Autodesk Fusion 360 part; units mm, degrees
note: some values were not read from the file. Chosen so that the rebuilt part matches the saved one: which bodies a step acts on. Set by a fixed rule: which sketch regions a step uses.
(part 4 of 6)
  spline S102 degree 5 poles (-98.784, -81.1032) (-98.7935, -81.0533) (-98.8123, -80.9538) (-98.8398, -80.8052) (-98.8751, -80.6086) (-98.9171, -80.3651) (-98.9568, -80.1241) (-98.9941, -79.8857) (-99.0292, -79.6497) (-99.062, -79.4165) (-99.0924, -79.1859) (-99.1207, -78.9582) (-99.1467, -78.7334) (-99.1706, -78.5115) (-99.1924, -78.2927) (-99.2121, -78.077) (-99.2297, -77.8644) (-99.2453, -77.6552) (-99.2589, -77.4492) (-99.2705, -77.2468) (-99.2802, -77.048) (-99.2881, -76.8529) (-99.2941, -76.6618) (-99.2983, -76.4747) (-99.3008, -76.2918) (-99.3016, -76.113) (-99.301, -75.9732) (-99.2997, -75.8702) (-99.2986, -75.8023) (-99.2979, -75.7686) knots 0 0 0 0 0 0 0.04 0.08 0.12 0.16 0.2 0.24 0.28 0.32 0.36 0.4 0.44 0.48 0.52 0.56 0.6 0.64 0.68 0.72 0.76 0.8 0.84 0.88 0.92 0.96 1 1 1 1 1 1
  arc A102 (-99.2979, -75.7686) -> (-97.2516, -81.4429) centre (-96.9333, -78.1219) ccw
  spline S103 degree 5 poles (-97.2516, -81.4429) (-97.2219, -81.4017) (-97.1628, -81.3194) (-97.0751, -81.1964) (-96.96, -81.0331) (-96.8191, -80.8302) (-96.6813, -80.6286) (-96.5466, -80.4283) (-96.4151, -80.2293) (-96.2868, -80.0317) (-96.1618, -79.8356) (-96.0399, -79.6412) (-95.9213, -79.4484) (-95.8059, -79.2574) (-95.6937, -79.0683) (-95.5847, -78.8812) (-95.4789, -78.696) (-95.3763, -78.5129) (-95.277, -78.332) (-95.1809, -78.1534) (-95.088, -77.9773) (-94.9985, -77.8039) (-94.9123, -77.6332) (-94.8294, -77.4655) (-94.7498, -77.3007) (-94.6735, -77.139) (-94.615, -77.012) (-94.5726, -76.9181) (-94.545, -76.8561) (-94.5313, -76.8253) knots 0 0 0 0 0 0 0.04 0.08 0.12 0.16 0.2 0.24 0.28 0.32 0.36 0.4 0.44 0.48 0.52 0.56 0.6 0.64 0.68 0.72 0.76 0.8 0.84 0.88 0.92 0.96 1 1 1 1 1 1
  arc A103 (-91.6439, -82.4317) -> (-94.5313, -76.8253) centre (-94.7025, -80.4602) ccw
  spline S104 degree 5 poles (-91.6439, -82.4317) (-91.6577, -82.3828) (-91.6851, -82.2853) (-91.7255, -82.1397) (-91.7778, -81.9469) (-91.8408, -81.708) (-91.9013, -81.4714) (-91.9594, -81.2371) (-92.0149, -81.0051) (-92.0678, -80.7756) (-92.1183, -80.5486) (-92.1663, -80.3242) (-92.2118, -80.1025) (-92.255, -79.8836) (-92.2957, -79.6675) (-92.3341, -79.4543) (-92.3702, -79.2441) (-92.404, -79.037) (-92.4355, -78.8331) (-92.4647, -78.6324) (-92.4917, -78.4351) (-92.5165, -78.2415) (-92.5391, -78.0517) (-92.5596, -77.8657) (-92.5781, -77.6836) (-92.5945, -77.5056) (-92.606, -77.3663) (-92.6138, -77.2635) (-92.6186, -77.1958) (-92.6208, -77.1622) knots 0 0 0 0 0 0 0.04 0.08 0.12 0.16 0.2 0.24 0.28 0.32 0.36 0.4 0.44 0.48 0.52 0.56 0.6 0.64 0.68 0.72 0.76 0.8 0.84 0.88 0.92 0.96 1 1 1 1 1 1
  arc A104 (-92.6208, -77.1622) -> (-90.0878, -82.6366) centre (-90.0601, -79.3005) ccw
  spline S105 degree 5 poles (-90.0878, -82.6366) (-90.0618, -82.5929) (-90.0101, -82.5058) (-89.9334, -82.3757) (-89.8329, -82.2029) (-89.7102, -81.9885) (-89.5905, -81.7757) (-89.4739, -81.5643) (-89.3602, -81.3546) (-89.2496, -81.1466) (-89.1422, -80.9404) (-89.0377, -80.7361) (-88.9363, -80.5337) (-88.838, -80.3334) (-88.7427, -80.1352) (-88.6504, -79.9393) (-88.5612, -79.7456) (-88.4749, -79.5543) (-88.3917, -79.3654) (-88.3116, -79.1791) (-88.2345, -78.9956) (-88.1604, -78.815) (-88.0894, -78.6375) (-88.0214, -78.4631) (-87.9565, -78.2921) (-87.8946, -78.1243) (-87.8474, -77.9927) (-87.8133, -77.8955) (-87.7912, -77.8314) (-87.7802, -77.7994) knots 0 0 0 0 0 0 0.04 0.08 0.12 0.16 0.2 0.24 0.28 0.32 0.36 0.4 0.44 0.48 0.52 0.56 0.6 0.64 0.68 0.72 0.76 0.8 0.84 0.88 0.92 0.96 1 1 1 1 1 1
  arc A105 (-84.4152, -83.1328) -> (-87.7802, -77.7994) centre (-87.634, -81.4354) ccw
  spline S106 degree 5 poles (-84.4152, -83.1328) (-84.4332, -83.0854) (-84.469, -82.9906) (-84.5219, -82.8491) (-84.5909, -82.6616) (-84.6744, -82.4291) (-84.7554, -82.1987) (-84.8336, -81.9703) (-84.9091, -81.7441) (-84.9818, -81.52) (-85.0519, -81.2983) (-85.1193, -81.0789) (-85.184, -80.862) (-85.246, -80.6477) (-85.3055, -80.436) (-85.3623, -80.227) (-85.4166, -80.0207) (-85.4683, -79.8173) (-85.5174, -79.6169) (-85.564, -79.4195) (-85.6081, -79.2254) (-85.6497, -79.0347) (-85.6888, -78.8475) (-85.7254, -78.664) (-85.7596, -78.4843) (-85.7915, -78.3083) (-85.8151, -78.1705) (-85.8318, -78.0689) (-85.8425, -78.0018) (-85.8477, -77.9685) knots 0 0 0 0 0 0 0.04 0.08 0.12 0.16 0.2 0.24 0.28 0.32 0.36 0.4 0.44 0.48 0.52 0.56 0.6 0.64 0.68 0.72 0.76 0.8 0.84 0.88 0.92 0.96 1 1 1 1 1 1
  arc A106 (-85.8477, -77.9685) -> (-82.8471, -83.2013) centre (-83.1103, -79.8755) ccw
  spline S107 degree 5 poles (-82.8471, -83.2013) (-82.825, -83.1556) (-82.7811, -83.0643) (-82.7161, -82.9279) (-82.631, -82.7471) (-82.5275, -82.5228) (-82.4268, -82.3003) (-82.329, -82.0797) (-82.2341, -81.8609) (-82.1421, -81.644) (-82.0529, -81.4292) (-81.9667, -81.2166) (-81.8834, -81.0061) (-81.8029, -80.798) (-81.7252, -80.5923) (-81.6503, -80.389) (-81.5783, -80.1883) (-81.5091, -79.9902) (-81.4426, -79.7948) (-81.379, -79.6022) (-81.3182, -79.4127) (-81.2602, -79.2263) (-81.2049, -79.0433) (-81.1524, -78.8637) (-81.1026, -78.6876) (-81.0555, -78.5151) (-81.02, -78.3799) (-80.9945, -78.2801) (-80.9781, -78.2142) (-80.97, -78.1815) knots 0 0 0 0 0 0 0.04 0.08 0.12 0.16 0.2 0.24 0.28 0.32 0.36 0.4 0.44 0.48 0.52 0.56 0.6 0.64 0.68 0.72 0.76 0.8 0.84 0.88 0.92 0.96 1 1 1 1 1 1
  arc A107 (-77.1529, -83.2013) -> (-80.97, -78.1815) centre (-80.5074, -81.7909) ccw
  spline S108 degree 5 poles (-77.1529, -83.2013) (-77.175, -83.1556) (-77.2189, -83.0643) (-77.2839, -82.9279) (-77.369, -82.7471) (-77.4725, -82.5228) (-77.5732, -82.3003) (-77.671, -82.0797) (-77.7659, -81.8609) (-77.8579, -81.644) (-77.9471, -81.4292) (-78.0333, -81.2166) (-78.1166, -81.0061) (-78.1971, -80.798) (-78.2748, -80.5923) (-78.3497, -80.389) (-78.4217, -80.1883) (-78.4909, -79.9902) (-78.5574, -79.7948) (-78.621, -79.6022) (-78.6818, -79.4127) (-78.7398, -79.2263) (-78.7951, -79.0433) (-78.8476, -78.8637) (-78.8974, -78.6876) (-78.9445, -78.5151) (-78.98, -78.3799) (-79.0055, -78.2801) (-79.0219, -78.2142) (-79.03, -78.1815) knots 0 0 0 0 0 0 0.04 0.08 0.12 0.16 0.2 0.24 0.28 0.32 0.36 0.4 0.44 0.48 0.52 0.56 0.6 0.64 0.68 0.72 0.76 0.8 0.84 0.88 0.92 0.96 1 1 1 1 1 1
  arc A108 (-79.03, -78.1815) -> (-75.5848, -83.1328) centre (-76.1369, -79.8427) ccw
  spline S109 degree 5 poles (-75.5848, -83.1328) (-75.5668, -83.0854) (-75.531, -82.9906) (-75.4781, -82.8491) (-75.4091, -82.6616) (-75.3256, -82.4291) (-75.2446, -82.1987) (-75.1664, -81.9703) (-75.0909, -81.7441) (-75.0182, -81.52) (-74.9481, -81.2983) (-74.8807, -81.0789) (-74.816, -80.862) (-74.754, -80.6477) (-74.6945, -80.436) (-74.6377, -80.227) (-74.5834, -80.0207) (-74.5317, -79.8173) (-74.4826, -79.6169) (-74.436, -79.4195) (-74.3919, -79.2254) (-74.3503, -79.0347) (-74.3112, -78.8475) (-74.2746, -78.664) (-74.2404, -78.4843) (-74.2085, -78.3083) (-74.1849, -78.1705) (-74.1682, -78.0689) (-74.1575, -78.0018) (-74.1523, -77.9685) knots 0 0 0 0 0 0 0.04 0.08 0.12 0.16 0.2 0.24 0.28 0.32 0.36 0.4 0.44 0.48 0.52 0.56 0.6 0.64 0.68 0.72 0.76 0.8 0.84 0.88 0.92 0.96 1 1 1 1 1 1
  arc A109 (-69.9122, -82.6366) -> (-74.1523, -77.9685) centre (-73.3769, -81.5239) ccw
  spline S110 degree 5 poles (-69.9122, -82.6366) (-69.9382, -82.5929) (-69.9899, -82.5058) (-70.0666, -82.3757) (-70.1671, -82.2029) (-70.2898, -81.9885) (-70.4095, -81.7757) (-70.5261, -81.5643) (-70.6398, -81.3546) (-70.7504, -81.1466) (-70.8578, -80.9404) (-70.9623, -80.7361) (-71.0637, -80.5337) (-71.162, -80.3334) (-71.2573, -80.1352) (-71.3496, -79.9393) (-71.4388, -79.7456) (-71.5251, -79.5543) (-71.6083, -79.3654) (-71.6884, -79.1791) (-71.7655, -78.9956) (-71.8396, -78.815) (-71.9106, -78.6375) (-71.9786, -78.4631) (-72.0435, -78.2921) (-72.1054, -78.1243) (-72.1526, -77.9927) (-72.1867, -77.8955) (-72.2088, -77.8314) (-72.2198, -77.7994) knots 0 0 0 0 0 0 0.04 0.08 0.12 0.16 0.2 0.24 0.28 0.32 0.36 0.4 0.44 0.48 0.52 0.56 0.6 0.64 0.68 0.72 0.76 0.8 0.84 0.88 0.92 0.96 1 1 1 1 1 1
  arc A110 (-72.2198, -77.7994) -> (-68.3561, -82.4317) centre (-69.1928, -79.2021) ccw
  spline S111 degree 5 poles (-68.3561, -82.4317) (-68.3423, -82.3828) (-68.3149, -82.2853) (-68.2745, -82.1397) (-68.2222, -81.9469) (-68.1592, -81.708) (-68.0987, -81.4714) (-68.0406, -81.2371) (-67.9851, -81.0051) (-67.9322, -80.7756) (-67.8817, -80.5486) (-67.8337, -80.3242) (-67.7882, -80.1025) (-67.745, -79.8836) (-67.7043, -79.6675) (-67.6659, -79.4543) (-67.6298, -79.2441) (-67.596, -79.037) (-67.5645, -78.8331) (-67.5353, -78.6324) (-67.5083, -78.4351) (-67.4835, -78.2415) (-67.4609, -78.0517) (-67.4404, -77.8657) (-67.4219, -77.6836) (-67.4055, -77.5056) (-67.394, -77.3663) (-67.3862, -77.2635) (-67.3814, -77.1958) (-67.3792, -77.1622) knots 0 0 0 0 0 0 0.04 0.08 0.12 0.16 0.2 0.24 0.28 0.32 0.36 0.4 0.44 0.48 0.52 0.56 0.6 0.64 0.68 0.72 0.76 0.8 0.84 0.88 0.92 0.96 1 1 1 1 1 1
  arc A111 (-62.7484, -81.4429) -> (-67.3792, -77.1622) centre (-66.2968, -80.6364) ccw
  spline S112 degree 5 poles (-62.7484, -81.4429) (-62.7781, -81.4017) (-62.8372, -81.3194) (-62.9249, -81.1964) (-63.04, -81.0331) (-63.1809, -80.8302) (-63.3187, -80.6286) (-63.4534, -80.4283) (-63.5849, -80.2293) (-63.7132, -80.0317) (-63.8382, -79.8356) (-63.9601, -79.6412) (-64.0787, -79.4484) (-64.1941, -79.2574) (-64.3063, -79.0683) (-64.4153, -78.8812) (-64.5211, -78.696) (-64.6237, -78.5129) (-64.723, -78.332) (-64.8191, -78.1534) (-64.912, -77.9773) (-65.0015, -77.8039) (-65.0877, -77.6332) (-65.1706, -77.4655) (-65.2502, -77.3007) (-65.3265, -77.139) (-65.385, -77.012) (-65.4274, -76.9181) (-65.455, -76.8561) (-65.4687, -76.8253) knots 0 0 0 0 0 0 0.04 0.08 0.12 0.16 0.2 0.24 0.28 0.32 0.36 0.4 0.44 0.48 0.52 0.56 0.6 0.64 0.68 0.72 0.76 0.8 0.84 0.88 0.92 0.96 1 1 1 1 1 1
  arc A112 (-65.4687, -76.8253) -> (-61.216, -81.1032) centre (-62.331, -77.9589) ccw
  spline S113 degree 5 poles (-61.216, -81.1032) (-61.2065, -81.0533) (-61.1877, -80.9538) (-61.1602, -80.8052) (-61.1249, -80.6086) (-61.0829, -80.3651) (-61.0432, -80.1241) (-61.0059, -79.8857) (-60.9708, -79.6497) (-60.938, -79.4165) (-60.9076, -79.1859) (-60.8793, -78.9582) (-60.8533, -78.7334) (-60.8294, -78.5115) (-60.8076, -78.2927) (-60.7879, -78.077) (-60.7703, -77.8644) (-60.7547, -77.6552) (-60.7411, -77.4492) (-60.7295, -77.2468) (-60.7198, -77.048) (-60.7119, -76.8529) (-60.7059, -76.6618) (-60.7017, -76.4747) (-60.6992, -76.2918) (-60.6984, -76.113) (-60.699, -75.9732) (-60.7003, -75.8702) (-60.7014, -75.8023) (-60.7021, -75.7686) knots 0 0 0 0 0 0 0.04 0.08 0.12 0.16 0.2 0.24 0.28 0.32 0.36 0.4 0.44 0.48 0.52 0.56 0.6 0.64 0.68 0.72 0.76 0.8 0.84 0.88 0.92 0.96 1 1 1 1 1 1
  arc A113 (-55.7158, -79.6294) -> (-60.7021, -75.7686) centre (-59.321, -79.1352) ccw
  spline S114 degree 5 poles (-55.7158, -79.6294) (-55.749, -79.591) (-55.815, -79.5142) (-55.9131, -79.3993) (-56.0421, -79.2466) (-56.2001, -79.0568) (-56.355, -78.8679) (-56.5066, -78.6801) (-56.6549, -78.4933) (-56.7999, -78.3077) (-56.9416, -78.1232) (-57.0799, -77.9401) (-57.2149, -77.7584) (-57.3465, -77.5783) (-57.4748, -77.3997) (-57.5997, -77.2227) (-57.7212, -77.0475) (-57.8394, -76.874) (-57.9541, -76.7025) (-58.0654, -76.533) (-58.1732, -76.3656) (-58.2775, -76.2006) (-58.3782, -76.0381) (-58.4754, -75.8782) (-58.5691, -75.721) (-58.6592, -75.5666) (-58.7285, -75.4452) (-58.779, -75.3553) (-58.8119, -75.296) (-58.8282, -75.2665) knots 0 0 0 0 0 0 0.04 0.08 0.12 0.16 0.2 0.24 0.28 0.32 0.36 0.4 0.44 0.48 0.52 0.56 0.6 0.64 0.68 0.72 0.76 0.8 0.84 0.88 0.92 0.96 1 1 1 1 1 1
  arc A114 (-58.8282, -75.2665) -> (-54.2189, -79.1574) centre (-55.6037, -76.1222) ccw
  spline S115 degree 5 poles (-54.2189, -79.1574) (-54.2138, -79.1069) (-54.2037, -79.0061) (-54.1893, -78.8557) (-54.1712, -78.6567) (-54.1506, -78.4106) (-54.1321, -78.167) (-54.1157, -77.9262) (-54.1013, -77.6881) (-54.089, -77.4529) (-54.0787, -77.2206) (-54.0704, -76.9913) (-54.0641, -76.765) (-54.0596, -76.5419) (-54.057, -76.322) (-54.0561, -76.1054) (-54.0571, -75.8922) (-54.0598, -75.6823) (-54.0642, -75.476) (-54.0703, -75.2733) (-54.078, -75.0744) (-54.0872, -74.8794) (-54.0979, -74.6885) (-54.1099, -74.5018) (-54.1234, -74.3193) (-54.1381, -74.1411) (-54.151, -74.0019) (-54.1612, -73.8994) (-54.1682, -73.8319) (-54.1718, -73.7983) knots 0 0 0 0 0 0 0.04 0.08 0.12 0.16 0.2 0.24 0.28 0.32 0.36 0.4 0.44 0.48 0.52 0.56 0.6 0.64 0.68 0.72 0.76 0.8 0.84 0.88 0.92 0.96 1 1 1 1 1 1
  arc A115 (-48.8681, -77.2099) -> (-54.1718, -73.7983) centre (-52.5026, -77.0318) ccw
  spline S116 degree 5 poles (-48.8681, -77.2099) (-48.9045, -77.1745) (-48.9769, -77.1037) (-49.0847, -76.9978) (-49.2264, -76.857) (-49.4004, -76.6816) (-49.5712, -76.507) (-49.7386, -76.3331) (-49.9026, -76.1599) (-50.0632, -75.9876) (-50.2204, -75.8163) (-50.3742, -75.6459) (-50.5245, -75.4767) (-50.6713, -75.3087) (-50.8147, -75.1419) (-50.9545, -74.9765) (-51.0909, -74.8125) (-51.2237, -74.6501) (-51.3529, -74.4892) (-51.4786, -74.33) (-51.6006, -74.1727) (-51.7188, -74.0174) (-51.8334, -73.8643) (-51.9441, -73.7135) (-52.0511, -73.5651) (-52.1544, -73.419) (-52.234, -73.3042) (-52.2921, -73.2191) (-52.3301, -73.1628) (-52.3489, -73.1348) knots 0 0 0 0 0 0 0.04 0.08 0.12 0.16 0.2 0.24 0.28 0.32 0.36 0.4 0.44 0.48 0.52 0.56 0.6 0.64 0.68 0.72 0.76 0.8 0.84 0.88 0.92 0.96 1 1 1 1 1 1
  arc A116 (-52.3489, -73.1348) -> (-47.418, -76.6092) centre (-49.062, -73.7063) ccw
  spline S117 degree 5 poles (-47.418, -76.6092) (-47.4173, -76.5585) (-47.4161, -76.4572) (-47.4148, -76.3061) (-47.4141, -76.1063) (-47.415, -75.8593) (-47.4178, -75.6151) (-47.4224, -75.3737) (-47.4289, -75.1353) (-47.4371, -74.8999) (-47.4471, -74.6675) (-47.4589, -74.4384) (-47.4722, -74.2124) (-47.4872, -73.9898) (-47.5038, -73.7705) (-47.5218, -73.5547) (-47.5414, -73.3423) (-47.5624, -73.1335) (-47.5847, -72.9283) (-47.6085, -72.7269) (-47.6334, -72.5294) (-47.6596, -72.336) (-47.6869, -72.1468) (-47.7152, -71.9618) (-47.7445, -71.7812) (-47.7747, -71.6049) (-47.7997, -71.4674) (-47.8188, -71.3661) (-47.8317, -71.2995) (-47.8382, -71.2664) knots 0 0 0 0 0 0 0.04 0.08 0.12 0.16 0.2 0.24 0.28 0.32 0.36 0.4 0.44 0.48 0.52 0.56 0.6 0.64 0.68 0.72 0.76 0.8 0.84 0.88 0.92 0.96 1 1 1 1 1 1
  arc A117 (-42.2572, -74.2027) -> (-47.8382, -71.2664) centre (-45.8935, -74.3421) ccw
  spline S118 degree 5 poles (-42.2572, -74.2027) (-42.2966, -74.1706) (-42.3749, -74.1065) (-42.4915, -74.0104) (-42.645, -73.8824) (-42.8336, -73.7229) (-43.0189, -73.5638) (-43.2008, -73.4052) (-43.3793, -73.247) (-43.5544, -73.0893) (-43.7259, -72.9323) (-43.894, -72.776) (-44.0584, -72.6205) (-44.2193, -72.4659) (-44.3767, -72.3123) (-44.5304, -72.1597) (-44.6805, -72.0083) (-44.827, -71.858) (-44.9698, -71.709) (-45.1088, -71.5613) (-45.244, -71.4153) (-45.3754, -71.2709) (-45.5029, -71.1283) (-45.6263, -70.9877) (-45.7459, -70.8492) (-45.8614, -70.7127) (-45.9508, -70.6052) (-46.0161, -70.5255) (-46.0588, -70.4728) (-46.08, -70.4466) knots 0 0 0 0 0 0 0.04 0.08 0.12 0.16 0.2 0.24 0.28 0.32 0.36 0.4 0.44 0.48 0.52 0.56 0.6 0.64 0.68 0.72 0.76 0.8 0.84 0.88 0.92 0.96 1 1 1 1 1 1
  arc A118 (-46.08, -70.4466) -> (-40.865, -73.478) centre (-42.7558, -70.7294) ccw
  spline S119 degree 5 poles (-40.865, -73.478) (-40.8688, -73.4274) (-40.8764, -73.3264) (-40.8882, -73.1757) (-40.905, -72.9766) (-40.9275, -72.7306) (-40.9515, -72.4876) (-40.9771, -72.2476) (-41.0043, -72.0106) (-41.0331, -71.7768) (-41.0633, -71.5462) (-41.095, -71.319) (-41.128, -71.095) (-41.1623, -70.8746) (-41.1979, -70.6576) (-41.2347, -70.4441) (-41.2727, -70.2343) (-41.3118, -70.0281) (-41.352, -69.8256) (-41.3931, -69.6271) (-41.4352, -69.4325) (-41.4782, -69.2421) (-41.5218, -69.0559) (-41.5662, -68.8742) (-41.6111, -68.6968) (-41.6566, -68.5238) (-41.6934, -68.389) (-41.7212, -68.2898) (-41.7399, -68.2245) (-41.7493, -68.1921) knots 0 0 0 0 0 0 0.04 0.08 0.12 0.16 0.2 0.24 0.28 0.32 0.36 0.4 0.44 0.48 0.52 0.56 0.6 0.64 0.68 0.72 0.76 0.8 0.84 0.88 0.92 0.96 1 1 1 1 1 1
  arc A119 (-35.9337, -70.6309) -> (-41.7493, -68.1921) centre (-39.5439, -71.0867) ccw
  spline S120 degree 5 poles (-35.9337, -70.6309) (-35.9757, -70.6023) (-36.0593, -70.5452) (-36.1838, -70.4597) (-36.3479, -70.3456) (-36.5497, -70.2031) (-36.7481, -70.0608) (-36.9432, -69.9186) (-37.1348, -69.7765) (-37.3229, -69.6348) (-37.5075, -69.4933) (-37.6885, -69.3522) (-37.8659, -69.2117) (-38.0397, -69.0717) (-38.2098, -68.9324) (-38.3763, -68.7938) (-38.539, -68.656) (-38.698, -68.519) (-38.8532, -68.383) (-39.0046, -68.2481) (-39.1521, -68.1143) (-39.2955, -67.9819) (-39.4349, -67.851) (-39.5701, -67.7217) (-39.7013, -67.5942) (-39.8283, -67.4683) (-39.9267, -67.369) (-39.9987, -67.2953) (-40.0459, -67.2465) (-40.0692, -67.2222) knots 0 0 0 0 0 0 0.04 0.08 0.12 0.16 0.2 0.24 0.28 0.32 0.36 0.4 0.44 0.48 0.52 0.56 0.6 0.64 0.68 0.72 0.76 0.8 0.84 0.88 0.92 0.96 1 1 1 1 1 1
  arc A120 (-40.0692, -67.2222) -> (-34.6099, -69.7876) centre (-36.7331, -67.2142) ccw
  spline S121 degree 5 poles (-34.6099, -69.7876) (-34.6181, -69.7374) (-34.6344, -69.6375) (-34.6594, -69.4885) (-34.6934, -69.2916) (-34.7373, -69.0485) (-34.7824, -68.8085) (-34.8289, -68.5716) (-34.8766, -68.3379) (-34.9256, -68.1075) (-34.9758, -67.8804) (-35.0271, -67.6568) (-35.0796, -67.4366) (-35.133, -67.2199) (-35.1874, -67.0069) (-35.2426, -66.7974) (-35.2987, -66.5917) (-35.3557, -66.3897) (-35.4133, -66.1915) (-35.4717, -65.9973) (-35.5306, -65.8072) (-35.5899, -65.6212) (-35.6496, -65.4396) (-35.7096, -65.2623) (-35.7699, -65.0896) (-35.8302, -64.9212) (-35.8787, -64.7901) (-35.9151, -64.6937) (-35.9393, -64.6303) (-35.9515, -64.5989) knots 0 0 0 0 0 0 0.04 0.08 0.12 0.16 0.2 0.24 0.28 0.32 0.36 0.4 0.44 0.48 0.52 0.56 0.6 0.64 0.68 0.72 0.76 0.8 0.84 0.88 0.92 0.96 1 1 1 1 1 1
  arc A121 (-29.9455, -66.5215) -> (-35.9515, -64.5989) centre (-33.5023, -67.2902) ccw
  spline S122 degree 5 poles (-29.9455, -66.5215) (-29.9898, -66.4967) (-30.0781, -66.4471) (-30.2096, -66.3727) (-30.383, -66.2734) (-30.5964, -66.149) (-30.8065, -66.0245) (-31.0132, -65.8999) (-31.2165, -65.7751) (-31.4162, -65.6502) (-31.6125, -65.5254) (-31.8051, -65.4006) (-31.994, -65.2761) (-32.1794, -65.1518) (-32.361, -65.0278) (-32.5389, -64.9042) (-32.713, -64.7811) (-32.8834, -64.6586) (-33.0498, -64.5366) (-33.2124, -64.4154) (-33.3709, -64.295) (-33.5254, -64.1756) (-33.6756, -64.0574) (-33.8217, -63.9404) (-33.9634, -63.8247) (-34.1009, -63.7104) (-34.2076, -63.62) (-34.2857, -63.5529) (-34.337, -63.5084) (-34.3624, -63.4862) knots 0 0 0 0 0 0 0.04 0.08 0.12 0.16 0.2 0.24 0.28 0.32 0.36 0.4 0.44 0.48 0.52 0.56 0.6 0.64 0.68 0.72 0.76 0.8 0.84 0.88 0.92 0.96 1 1 1 1 1 1
  arc A122 (-34.3624, -63.4862) -> (-28.7003, -65.566) centre (-31.0396, -63.1875) ccw
  spline S123 degree 5 poles (-28.7003, -65.566) (-28.7127, -65.5168) (-28.7378, -65.4186) (-28.7756, -65.2724) (-28.8267, -65.0792) (-28.8915, -64.8408) (-28.9574, -64.6057) (-29.0243, -64.3737) (-29.0923, -64.1451) (-29.1612, -63.9198) (-29.231, -63.698) (-29.3016, -63.4797) (-29.373, -63.2649) (-29.4451, -63.0537) (-29.5179, -62.8462) (-29.5912, -62.6424) (-29.665, -62.4423) (-29.7393, -62.2461) (-29.814, -62.0537) (-29.8891, -61.8653) (-29.9643, -61.681) (-30.0396, -61.5009) (-30.115, -61.3252) (-30.1902, -61.1538) (-30.2652, -60.987) (-30.3401, -60.8245) (-30.3997, -60.6981) (-30.4444, -60.6053) (-30.4741, -60.5443) (-30.489, -60.514) knots 0 0 0 0 0 0 0.04 0.08 0.12 0.16 0.2 0.24 0.28 0.32 0.36 0.4 0.44 0.48 0.52 0.56 0.6 0.64 0.68 0.72 0.76 0.8 0.84 0.88 0.92 0.96 1 1 1 1 1 1
  arc A123 (-24.3382, -61.9058) -> (-30.489, -60.514) centre (-27.8145, -62.9816) ccw
  spline S124 degree 5 poles (-24.3382, -61.9058) (-24.3845, -61.885) (-24.4768, -61.8433) (-24.6143, -61.7806) (-24.7957, -61.6968) (-25.0191, -61.5915) (-25.2393, -61.4858) (-25.4561, -61.3796) (-25.6695, -61.273) (-25.8793, -61.1661) (-26.0857, -61.0588) (-26.2884, -60.9513) (-26.4875, -60.8437) (-26.683, -60.736) (-26.8747, -60.6283) (-27.0627, -60.5207) (-27.2469, -60.4133) (-27.4273, -60.306) (-27.6038, -60.199) (-27.7763, -60.0924) (-27.9447, -59.9863) (-28.109, -59.8809) (-28.2689, -59.7762) (-28.4246, -59.6723) (-28.5759, -59.5695) (-28.7229, -59.4676) (-28.837, -59.3868) (-28.9207, -59.3268) (-28.9756, -59.2869) (-29.0029, -59.267) knots 0 0 0 0 0 0 0.04 0.08 0.12 0.16 0.2 0.24 0.28 0.32 0.36 0.4 0.44 0.48 0.52 0.56 0.6 0.64 0.68 0.72 0.76 0.8 0.84 0.88 0.92 0.96 1 1 1 1 1 1
  arc A124 (-29.0029, -59.267) -> (-23.181, -60.8454) centre (-25.7188, -58.6799) ccw
  spline S125 degree 5 poles (-23.181, -60.8454) (-23.1977, -60.7975) (-23.2312, -60.7019) (-23.2817, -60.5595) (-23.3494, -60.3715) (-23.4348, -60.1397) (-23.5209, -59.9112) (-23.6078, -59.6859) (-23.6954, -59.4641) (-23.7836, -59.2457) (-23.8725, -59.0308) (-23.9619, -58.8195) (-24.0518, -58.6117) (-24.142, -58.4076) (-24.2325, -58.2072) (-24.3233, -58.0106) (-24.4143, -57.8177) (-24.5055, -57.6287) (-24.5967, -57.4436) (-24.6878, -57.2624) (-24.7789, -57.0854) (-24.8696, -56.9125) (-24.96, -56.744) (-25.0498, -56.5799) (-25.1391, -56.4202) (-25.2278, -56.2649) (-25.2983, -56.1442) (-25.3509, -56.0556) (-25.3858, -55.9974) (-25.4032, -55.9685) knots 0 0 0 0 0 0 0.04 0.08 0.12 0.16 0.2 0.24 0.28 0.32 0.36 0.4 0.44 0.48 0.52 0.56 0.6 0.64 0.68 0.72 0.76 0.8 0.84 0.88 0.92 0.96 1 1 1 1 1 1
  arc A125 (-19.1546, -56.819) -> (-25.4032, -55.9685) centre (-22.5239, -58.1936) ccw
  spline S126 degree 5 poles (-19.1546, -56.819) (-19.2025, -56.8023) (-19.2981, -56.7688) (-19.4405, -56.7183) (-19.6285, -56.6506) (-19.8603, -56.5652) (-20.0888, -56.4791) (-20.3141, -56.3922) (-20.5359, -56.3046) (-20.7543, -56.2164) (-20.9692, -56.1275) (-21.1805, -56.0381) (-21.3883, -55.9482) (-21.5924, -55.858) (-21.7928, -55.7675) (-21.9894, -55.6767) (-22.1823, -55.5857) (-22.3713, -55.4945) (-22.5564, -55.4033) (-22.7376, -55.3122) (-22.9146, -55.2211) (-23.0875, -55.1304) (-23.256, -55.04) (-23.4201, -54.9502) (-23.5798, -54.8609) (-23.7351, -54.7722) (-23.8558, -54.7017) (-23.9444, -54.6491) (-24.0026, -54.6142) (-24.0315, -54.5968) knots 0 0 0 0 0 0 0.04 0.08 0.12 0.16 0.2 0.24 0.28 0.32 0.36 0.4 0.44 0.48 0.52 0.56 0.6 0.64 0.68 0.72 0.76 0.8 0.84 0.88 0.92 0.96 1 1 1 1 1 1
  arc A126 (-24.0315, -54.5968) -> (-18.0942, -55.6618) centre (-20.8111, -53.7256) ccw
  spline S127 degree 5 poles (-18.0942, -55.6618) (-18.115, -55.6155) (-18.1567, -55.5232) (-18.2194, -55.3857) (-18.3032, -55.2043) (-18.4085, -54.9809) (-18.5142, -54.7607) (-18.6204, -54.5439) (-18.727, -54.3305) (-18.8339, -54.1207) (-18.9412, -53.9143) (-19.0487, -53.7116) (-19.1563, -53.5125) (-19.264, -53.317) (-19.3717, -53.1253) (-19.4793, -52.9373) (-19.5867, -52.7531) (-19.694, -52.5727) (-19.801, -52.3962) (-19.9076, -52.2237) (-20.0137, -52.0553) (-20.1191, -51.891) (-20.2238, -51.7311) (-20.3277, -51.5754) (-20.4305, -51.4241) (-20.5324, -51.2771) (-20.6132, -51.163) (-20.6732, -51.0793) (-20.7131, -51.0244) (-20.733, -50.9971) knots 0 0 0 0 0 0 0.04 0.08 0.12 0.16 0.2 0.24 0.28 0.32 0.36 0.4 0.44 0.48 0.52 0.56 0.6 0.64 0.68 0.72 0.76 0.8 0.84 0.88 0.92 0.96 1 1 1 1 1 1
  arc A127 (-14.434, -51.2997) -> (-20.733, -50.9971) centre (-17.6707, -52.9628) ccw
  spline S128 degree 5 poles (-14.434, -51.2997) (-14.4832, -51.2873) (-14.5814, -51.2622) (-14.7276, -51.2244) (-14.9208, -51.1733) (-15.1592, -51.1085) (-15.3943, -51.0426) (-15.6263, -50.9757) (-15.8549, -50.9077) (-16.0802, -50.8388) (-16.302, -50.769) (-16.5203, -50.6984) (-16.7351, -50.627) (-16.9463, -50.5549) (-17.1538, -50.4821) (-17.3576, -50.4088) (-17.5577, -50.335) (-17.7539, -50.2607) (-17.9463, -50.186) (-18.1347, -50.1109) (-18.319, -50.0357) (-18.4991, -49.9604) (-18.6748, -49.885) (-18.8462, -49.8098) (-19.013, -49.7348) (-19.1755, -49.6599) (-19.3019, -49.6003) (-19.3947, -49.5556) (-19.4557, -49.5259) (-19.486, -49.511) knots 0 0 0 0 0 0 0.04 0.08 0.12 0.16 0.2 0.24 0.28 0.32 0.36 0.4 0.44 0.48 0.52 0.56 0.6 0.64 0.68 0.72 0.76 0.8 0.84 0.88 0.92 0.96 1 1 1 1 1 1
  arc A128 (-19.486, -49.511) -> (-13.4785, -50.0545) centre (-16.3538, -48.3625) ccw
  spline S129 degree 5 poles (-13.4785, -50.0545) (-13.5033, -50.0102) (-13.5529, -49.9219) (-13.6273, -49.7904) (-13.7266, -49.617) (-13.851, -49.4036) (-13.9755, -49.1935) (-14.1001, -48.9868) (-14.2249, -48.7835) (-14.3498, -48.5838) (-14.4746, -48.3875) (-14.5994, -48.1949) (-14.7239, -48.006) (-14.8482, -47.8206) (-14.9722, -47.639) (-15.0958, -47.4611) (-15.2189, -47.287) (-15.3414, -47.1166) (-15.4634, -46.9502) (-15.5846, -46.7876) (-15.705, -46.6291) (-15.8244, -46.4746) (-15.9426, -46.3244) (-16.0596, -46.1783) (-16.1753, -46.0366) (-16.2896, -45.8991) (-16.38, -45.7924) (-16.4471, -45.7143) (-16.4916, -45.663) (-16.5138, -45.6376) knots 0 0 0 0 0 0 0.04 0.08 0.12 0.16 0.2 0.24 0.28 0.32 0.36 0.4 0.44 0.48 0.52 0.56 0.6 0.64 0.68 0.72 0.76 0.8 0.84 0.88 0.92 0.96 1 1 1 1 1 1
  arc A129 (-10.2124, -45.3901) -> (-16.5138, -45.6376) centre (-13.2918, -47.3289) ccw
  spline S130 degree 5 poles (-10.2124, -45.3901) (-10.2626, -45.3819) (-10.3625, -45.3656) (-10.5115, -45.3406) (-10.7084, -45.3066) (-10.9515, -45.2627) (-11.1915, -45.2176) (-11.4284, -45.1711) (-11.6621, -45.1234) (-11.8925, -45.0744) (-12.1196, -45.0242) (-12.3432, -44.9729) (-12.5634, -44.9204) (-12.7801, -44.867) (-12.9931, -44.8126) (-13.2026, -44.7574) (-13.4083, -44.7013) (-13.6103, -44.6443) (-13.8085, -44.5867) (-14.0027, -44.5283) (-14.1928, -44.4694) (-14.3788, -44.4101) (-14.5604, -44.3504) (-14.7377, -44.2904) (-14.9104, -44.2301) (-15.0788, -44.1698) (-15.2099, -44.1213) (-15.3063, -44.0849) (-15.3697, -44.0607) (-15.4011, -44.0485) knots 0 0 0 0 0 0 0.04 0.08 0.12 0.16 0.2 0.24 0.28 0.32 0.36 0.4 0.44 0.48 0.52 0.56 0.6 0.64 0.68 0.72 0.76 0.8 0.84 0.88 0.92 0.96 1 1 1 1 1 1
  arc A130 (-15.4011, -44.0485) -> (-9.3691, -44.0663) centre (-12.3809, -42.6314) ccw
  spline S131 degree 5 poles (-9.3691, -44.0663) (-9.3977, -44.0243) (-9.4548, -43.9407) (-9.5403, -43.8162) (-9.6544, -43.6521) (-9.7969, -43.4503) (-9.9392, -43.2519) (-10.0814, -43.0568) (-10.2235, -42.8652) (-10.3652, -42.6771) (-10.5067, -42.4925) (-10.6478, -42.3115) (-10.7883, -42.1341) (-10.9283, -41.9603) (-11.0676, -41.7902) (-11.2062, -41.6237) (-11.344, -41.461) (-11.481, -41.302) (-11.617, -41.1468) (-11.7519, -40.9954) (-11.8857, -40.8479) (-12.0181, -40.7045) (-12.149, -40.5651) (-12.2783, -40.4299) (-12.4058, -40.2987) (-12.5317, -40.1717) (-12.631, -40.0733) (-12.7047, -40.0013) (-12.7535, -39.9541) (-12.7778, -39.9308) knots 0 0 0 0 0 0 0.04 0.08 0.12 0.16 0.2 0.24 0.28 0.32 0.36 0.4 0.44 0.48 0.52 0.56 0.6 0.64 0.68 0.72 0.76 0.8 0.84 0.88 0.92 0.96 1 1 1 1 1 1
  arc A131 (-6.522, -39.135) -> (-12.7778, -39.9308) centre (-9.4207, -41.3348) ccw
  spline S132 degree 5 poles (-6.522, -39.135) (-6.5726, -39.1312) (-6.6736, -39.1236) (-6.8243, -39.1118) (-7.0234, -39.095) (-7.2694, -39.0725) (-7.5124, -39.0485) (-7.7524, -39.0229) (-7.9894, -38.9957) (-8.2232, -38.9669) (-8.4538, -38.9367) (-8.681, -38.905) (-8.905, -38.872) (-9.1254, -38.8377) (-9.3424, -38.8021) (-9.5559, -38.7653) (-9.7657, -38.7273) (-9.9719, -38.6882) (-10.1744, -38.648) (-10.3729, -38.6069) (-10.5675, -38.5648) (-10.7579, -38.5218) (-10.9441, -38.4782) (-11.1258, -38.4338) (-11.3032, -38.3889) (-11.4762, -38.3434) (-11.611, -38.3066) (-11.7102, -38.2788) (-11.7755, -38.2601) (-11.8079, -38.2507) knots 0 0 0 0 0 0 0.04 0.08 0.12 0.16 0.2 0.24 0.28 0.32 0.36 0.4 0.44 0.48 0.52 0.56 0.6 0.64 0.68 0.72 0.76 0.8 0.84 0.88 0.92 0.96 1 1 1 1 1 1
  arc A132 (-11.8079, -38.2507) -> (-5.7973, -37.7428) centre (-8.9227, -36.5758) ccw
  spline S133 degree 5 poles (-5.7973, -37.7428) (-5.8294, -37.7034) (-5.8935, -37.6251) (-5.9896, -37.5085) (-6.1176, -37.355) (-6.2771, -37.1664) (-6.4362, -36.9811) (-6.5948, -36.7992) (-6.753, -36.6207) (-6.9107, -36.4456) (-7.0677, -36.2741) (-7.224, -36.106) (-7.3795, -35.9416) (-7.5341, -35.7807) (-7.6877, -35.6233) (-7.8403, -35.4696) (-7.9917, -35.3195) (-8.142, -35.173) (-8.291, -35.0302) (-8.4387, -34.8912) (-8.5847, -34.756) (-8.7291, -34.6246) (-8.8717, -34.4971) (-9.0123, -34.3737) (-9.1508, -34.2541) (-9.2873, -34.1386) (-9.3948, -34.0492) (-9.4745, -33.9839) (-9.5272, -33.9412) (-9.5534, -33.92) knots 0 0 0 0 0 0 0.04 0.08 0.12 0.16 0.2 0.24 0.28 0.32 0.36 0.4 0.44 0.48 0.52 0.56 0.6 0.64 0.68 0.72 0.76 0.8 0.84 0.88 0.92 0.96 1 1 1 1 1 1
  arc A133 (-3.3908, -32.582) -> (-9.5534, -33.92) centre (-6.0867, -35.0261) ccw
  spline S134 degree 5 poles (-3.3908, -32.582) (-3.4415, -32.5827) (-3.5428, -32.5839) (-3.6939, -32.5852) (-3.8937, -32.5859) (-4.1407, -32.585) (-4.3849, -32.5822) (-4.6263, -32.5776) (-4.8647, -32.5711) (-5.1001, -32.5629) (-5.3325, -32.5529) (-5.5616, -32.5411) (-5.7876, -32.5278) (-6.0102, -32.5128) (-6.2295, -32.4962) (-6.4453, -32.4782) (-6.6577, -32.4586) (-6.8665, -32.4376) (-7.0717, -32.4153) (-7.2731, -32.3915) (-7.4706, -32.3666) (-7.664, -32.3404) (-7.8532, -32.3131) (-8.0382, -32.2848) (-8.2188, -32.2555) (-8.3951, -32.2253) (-8.5326, -32.2003) (-8.6339, -32.1812) (-8.7005, -32.1683) (-8.7336, -32.1618) knots 0 0 0 0 0 0 0.04 0.08 0.12 0.16 0.2 0.24 0.28 0.32 0.36 0.4 0.44 0.48 0.52 0.56 0.6 0.64 0.68 0.72 0.76 0.8 0.84 0.88 0.92 0.96 1 1 1 1 1 1
  arc A134 (-8.7336, -32.1618) -> (-2.7901, -31.1319) centre (-6.0053, -30.2418) ccw
  spline S135 degree 5 poles (-2.7901, -31.1319) (-2.8255, -31.0955) (-2.8963, -31.0231) (-3.0022, -30.9153) (-3.143, -30.7736) (-3.3184, -30.5996) (-3.493, -30.4288) (-3.6669, -30.2614) (-3.8401, -30.0974) (-4.0124, -29.9368) (-4.1837, -29.7796) (-4.3541, -29.6258) (-4.5233, -29.4755) (-4.6913, -29.3287) (-4.8581, -29.1853) (-5.0235, -29.0455) (-5.1875, -28.9091) (-5.3499, -28.7763) (-5.5108, -28.6471) (-5.67, -28.5214) (-5.8273, -28.3994) (-5.9826, -28.2812) (-6.1357, -28.1666) (-6.2865, -28.0559) (-6.4349, -27.9489) (-6.581, -27.8456) (-6.6958, -27.766) (-6.7809, -27.7079) (-6.8372, -27.6699) (-6.8652, -27.6511) knots 0 0 0 0 0 0 0.04 0.08 0.12 0.16 0.2 0.24 0.28 0.32 0.36 0.4 0.44 0.48 0.52 0.56 0.6 0.64 0.68 0.72 0.76 0.8 0.84 0.88 0.92 0.96 1 1 1 1 1 1
  arc A135 (-0.8426, -25.7811) -> (-6.8652, -27.6511) centre (-3.3152, -28.4509) ccw
  spline S136 degree 5 poles (-0.8426, -25.7811) (-0.8931, -25.7862) (-0.9939, -25.7963) (-1.1443, -25.8107) (-1.3433, -25.8288) (-1.5894, -25.8494) (-1.833, -25.8679) (-2.0738, -25.8843) (-2.3119, -25.8987) (-2.5471, -25.911) (-2.7794, -25.9213) (-3.0087, -25.9296) (-3.235, -25.9359) (-3.4581, -25.9404) (-3.678, -25.943) (-3.8946, -25.9439) (-4.1078, -25.9429) (-4.3177, -25.9402) (-4.524, -25.9358) (-4.7267, -25.9297) (-4.9256, -25.922) (-5.1206, -25.9128) (-5.3115, -25.9021) (-5.4982, -25.8901) (-5.6807, -25.8766) (-5.8589, -25.8619) (-5.9981, -25.849) (-6.1006, -25.8388) (-6.1681, -25.8318) (-6.2017, -25.8282) knots 0 0 0 0 0 0 0.04 0.08 0.12 0.16 0.2 0.24 0.28 0.32 0.36 0.4 0.44 0.48 0.52 0.56 0.6 0.64 0.68 0.72 0.76 0.8 0.84 0.88 0.92 0.96 1 1 1 1 1 1
  arc A136 (-6.2017, -25.8282) -> (-0.3706, -24.2842) centre (-3.6512, -23.6776) ccw
  spline S137 degree 5 poles (-0.3706, -24.2842) (-0.409, -24.251) (-0.4858, -24.185) (-0.6007, -24.0869) (-0.7534, -23.9579) (-0.9432, -23.7999) (-1.1321, -23.645) (-1.3199, -23.4934) (-1.5067, -23.3451) (-1.6923, -23.2001) (-1.8768, -23.0584) (-2.0599, -22.9201) (-2.2416, -22.7851) (-2.4217, -22.6535) (-2.6003, -22.5252) (-2.7773, -22.4003) (-2.9525, -22.2788) (-3.126, -22.1606) (-3.2975, -22.0459) (-3.467, -21.9346) (-3.6344, -21.8268) (-3.7994, -21.7225) (-3.9619, -21.6218) (-4.1218, -21.5246) (-4.279, -21.4309) (-4.4334, -21.3408) (-4.5548, -21.2715) (-4.6447, -21.221) (-4.704, -21.1881) (-4.7335, -21.1718) knots 0 0 0 0 0 0 0.04 0.08 0.12 0.16 0.2 0.24 0.28 0.32 0.36 0.4 0.44 0.48 0.52 0.56 0.6 0.64 0.68 0.72 0.76 0.8 0.84 0.88 0.92 0.96 1 1 1 1 1 1
  arc A137 (1.1032, -18.784) -> (-4.7335, -21.1718) centre (-1.1274, -21.6591) ccw
  spline S138 degree 5 poles (1.1032, -18.784) (1.0533, -18.7935) (0.9538, -18.8123) (0.8052, -18.8398) (0.6086, -18.8751) (0.3651, -18.9171) (0.1241, -18.9568) (-0.1143, -18.9941) (-0.3503, -19.0292) (-0.5835, -19.062) (-0.8141, -19.0924) (-1.0418, -19.1207) (-1.2666, -19.1467) (-1.4885, -19.1706) (-1.7073, -19.1924) (-1.923, -19.2121) (-2.1356, -19.2297) (-2.3448, -19.2453) (-2.5508, -19.2589) (-2.7532, -19.2705) (-2.952, -19.2802) (-3.1471, -19.2881) (-3.3382, -19.2941) (-3.5253, -19.2983) (-3.7082, -19.3008) (-3.887, -19.3016) (-4.0268, -19.301) (-4.1298, -19.2997) (-4.1977, -19.2986) (-4.2314, -19.2979) knots 0 0 0 0 0 0 0.04 0.08 0.12 0.16 0.2 0.24 0.28 0.32 0.36 0.4 0.44 0.48 0.52 0.56 0.6 0.64 0.68 0.72 0.76 0.8 0.84 0.88 0.92 0.96 1 1 1 1 1 1
  arc A138 (-4.2314, -19.2979) -> (1.4429, -17.2516) centre (-1.8781, -16.9333) ccw
  spline S139 degree 5 poles (1.4429, -17.2516) (1.4017, -17.2219) (1.3194, -17.1628) (1.1964, -17.0751) (1.0331, -16.96) (0.8302, -16.8191) (0.6286, -16.6813) (0.4283, -16.5466) (0.2293, -16.4151) (0.0317, -16.2868) (-0.1644, -16.1618) (-0.3588, -16.0399) (-0.5516, -15.9213) (-0.7426, -15.8059) (-0.9317, -15.6937) (-1.1188, -15.5847) (-1.304, -15.4789) (-1.4871, -15.3763) (-1.668, -15.277) (-1.8466, -15.1809) (-2.0227, -15.088) (-2.1961, -14.9985) (-2.3668, -14.9123) (-2.5345, -14.8294) (-2.6993, -14.7498) (-2.861, -14.6735) (-2.988, -14.615) (-3.0819, -14.5726) (-3.1439, -14.545) (-3.1747, -14.5313) knots 0 0 0 0 0 0 0.04 0.08 0.12 0.16 0.2 0.24 0.28 0.32 0.36 0.4 0.44 0.48 0.52 0.56 0.6 0.64 0.68 0.72 0.76 0.8 0.84 0.88 0.92 0.96 1 1 1 1 1 1
  arc A139 (2.4317, -11.6439) -> (-3.1747, -14.5313) centre (0.4602, -14.7025) ccw
  spline S140 degree 5 poles (2.4317, -11.6439) (2.3828, -11.6577) (2.2853, -11.6851) (2.1397, -11.7255) (1.9469, -11.7778) (1.708, -11.8408) (1.4714, -11.9013) (1.2371, -11.9594) (1.0051, -12.0149) (0.7756, -12.0678) (0.5486, -12.1183) (0.3242, -12.1663) (0.1025, -12.2118) (-0.1164, -12.255) (-0.3325, -12.2957) (-0.5457, -12.3341) (-0.7559, -12.3702) (-0.963, -12.404) (-1.1669, -12.4355) (-1.3676, -12.4647) (-1.5649, -12.4917) (-1.7585, -12.5165) (-1.9483, -12.5391) (-2.1343, -12.5596) (-2.3164, -12.5781) (-2.4944, -12.5945) (-2.6337, -12.606) (-2.7365, -12.6138) (-2.8042, -12.6186) (-2.8378, -12.6208) knots 0 0 0 0 0 0 0.04 0.08 0.12 0.16 0.2 0.24 0.28 0.32 0.36 0.4 0.44 0.48 0.52 0.56 0.6 0.64 0.68 0.72 0.76 0.8 0.84 0.88 0.92 0.96 1 1 1 1 1 1
  arc A140 (-2.8378, -12.6208) -> (2.6366, -10.0878) centre (-0.6995, -10.0601) ccw
  spline S141 degree 5 poles (2.6366, -10.0878) (2.5929, -10.0618) (2.5058, -10.0101) (2.3757, -9.9334) (2.2029, -9.8329) (1.9885, -9.7102) (1.7757, -9.5905) (1.5643, -9.4739) (1.3546, -9.3602) (1.1466, -9.2496) (0.9404, -9.1422) (0.7361, -9.0377) (0.5337, -8.9363) (0.3334, -8.838) (0.1352, -8.7427) (-0.0607, -8.6504) (-0.2544, -8.5612) (-0.4457, -8.4749) (-0.6346, -8.3917) (-0.8209, -8.3116) (-1.0044, -8.2345) (-1.185, -8.1604) (-1.3625, -8.0894) (-1.5369, -8.0214) (-1.7079, -7.9565) (-1.8757, -7.8946) (-2.0073, -7.8474) (-2.1045, -7.8133) (-2.1686, -7.7912) (-2.2006, -7.7802) knots 0 0 0 0 0 0 0.04 0.08 0.12 0.16 0.2 0.24 0.28 0.32 0.36 0.4 0.44 0.48 0.52 0.56 0.6 0.64 0.68 0.72 0.76 0.8 0.84 0.88 0.92 0.96 1 1 1 1 1 1
  arc A141 (3.1328, -4.4152) -> (-2.2006, -7.7802) centre (1.4354, -7.634) ccw
  spline S142 degree 5 poles (3.1328, -4.4152) (3.0854, -4.4332) (2.9906, -4.469) (2.8491, -4.5219) (2.6616, -4.5909) (2.4291, -4.6744) (2.1987, -4.7554) (1.9703, -4.8336) (1.7441, -4.9091) (1.52, -4.9818) (1.2983, -5.0519) (1.0789, -5.1193) (0.862, -5.184) (0.6477, -5.246) (0.436, -5.3055) (0.227, -5.3623) (0.0207, -5.4166) (-0.1827, -5.4683) (-0.3831, -5.5174) (-0.5805, -5.564) (-0.7746, -5.6081) (-0.9653, -5.6497) (-1.1525, -5.6888) (-1.336, -5.7254) (-1.5157, -5.7596) (-1.6917, -5.7915) (-1.8295, -5.8151) (-1.9311, -5.8318) (-1.9982, -5.8425) (-2.0315, -5.8477) knots 0 0 0 0 0 0 0.04 0.08 0.12 0.16 0.2 0.24 0.28 0.32 0.36 0.4 0.44 0.48 0.52 0.56 0.6 0.64 0.68 0.72 0.76 0.8 0.84 0.88 0.92 0.96 1 1 1 1 1 1
  arc A142 (-2.0315, -5.8477) -> (3.2013, -2.8471) centre (-0.1245, -3.1103) ccw
  spline S143 degree 5 poles (3.2013, -2.8471) (3.1556, -2.825) (3.0643, -2.7811) (2.9279, -2.7161) (2.7471, -2.631) (2.5228, -2.5275) (2.3003, -2.4268) (2.0797, -2.329) (1.8609, -2.2341) (1.644, -2.1421) (1.4292, -2.0529) (1.2166, -1.9667) (1.0061, -1.8834) (0.798, -1.8029) (0.5923, -1.7252) (0.389, -1.6503) (0.1883, -1.5783) (-0.0098, -1.5091) (-0.2052, -1.4426) (-0.3978, -1.379) (-0.5873, -1.3182) (-0.7737, -1.2602) (-0.9567, -1.2049) (-1.1363, -1.1524) (-1.3124, -1.1026) (-1.4849, -1.0555) (-1.6201, -1.02) (-1.7199, -0.9945) (-1.7858, -0.9781) (-1.8185, -0.97) knots 0 0 0 0 0 0 0.04 0.08 0.12 0.16 0.2 0.24 0.28 0.32 0.36 0.4 0.44 0.48 0.52 0.56 0.6 0.64 0.68 0.72 0.76 0.8 0.84 0.88 0.92 0.96 1 1 1 1 1 1
  arc A143 (3.2013, 2.8471) -> (-1.8185, -0.97) centre (1.7909, -0.5074) ccw
  point P0 (1.9862, 2.2887)
  point P1 (0.8709, 1.8313)
  point P2 (-0.1386, 1.4655)
  point P3 (-1.0367, 1.1818)
  point P4 (1.8737, 4.8656)
  point P5 (0.7227, 5.224)
  point P6 (-0.3147, 5.5004)
  point P7 (-1.2341, 5.7048)
  point P8 (1.4747, 9.4256)
  point P9 (0.4035, 8.8727)
  point P10 (-0.5702, 8.4204)
  point P11 (-1.4401, 8.0594)
  point P12 (1.1381, 11.9828)
  point P13 (-0.0397, 12.2396)
  point P14 (-1.0974, 12.4245)
  point P15 (-2.0311, 12.548)
  point P16 (0.3432, 16.4907)
  point P17 (-0.6758, 15.8466)
  point P18 (-1.6063, 15.3111)
  point P19 (-2.4415, 14.8756)
  point P20 (-0.2151, 19.0089)
  point P21 (-1.4108, 19.162)
  point P22 (-2.4805, 19.254)
  point P23 (-3.4214, 19.2957)
  point P24 (-1.3998, 23.4303)
  point P25 (-2.3587, 22.6998)
  point P26 (-3.2391, 22.0853)
  point P27 (-4.0331, 21.5787)
  point P28 (-2.1754, 25.8902)
  point P29 (-3.3799, 25.9386)
  point P30 (-4.4536, 25.937)
  point P31 (-5.3945, 25.8966)
  point P32 (-3.741, 30.1916)
  point P33 (-4.6326, 29.3803)
  point P34 (-5.4561, 28.6914)
  point P35 (-6.2029, 28.1175)
  point P36 (-4.728, 32.5746)
  point P37 (-5.9322, 32.5178)